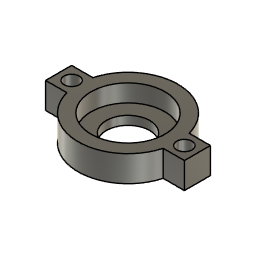
wind_direction (Autodesk Fusion 360 archive; units mm, degrees)
design "uchwyt lozysko"
Autodesk Fusion 360 part; units mm, degrees
sketch "Szkic1" plane through (0, 0, 0) normal (0, 0, 1) x (1, 0, 0)
  circle A0 centre (0, 0) radius 5
  circle A1 centre (0, 0) radius 8.5
  circle A2 centre (0, 0) radius 11.5
  circle A3 centre (13, 0) radius 1.75
  circle A4 centre (-13, 0) radius 1.75
  line L0 (16, 3) -> (-16, 3)
  line L1 (-16, 3) -> (-16, -3)
  line L2 (-16, -3) -> (16, -3)
  line L3 (16, -3) -> (16, 3)
  line L4 (16, 3) -> (-16, -3) construction
  line L5 (-16, 3) -> (16, -3) construction
  dimension "d1" = 10
  dimension "d2" = 17
  dimension "d3" = 23
  dimension "d4" = 3.5
  dimension "d5" = 13
  dimension "d6" = 3.5
  dimension "d7" = 13
  dimension "d8" = 32
  dimension "d9" = 6
  constraint coincident A0.centre A1.centre
  constraint concentric A0 A2
  constraint horizontal L0
  constraint perpendicular L0 L1
  constraint parallel L0 L2
  constraint parallel L1 L3
  constraint coincident L4 A0.centre
  constraint coincident L5 A0.centre
  constraint horizontal A0.centre A4.centre
  constraint horizontal A0.centre A3.centre
  measures "d1" diameter of A0
  measures "d2" diameter of A1
  measures "d3" diameter of A2
  measures "d4" diameter of A3
  measures "d5" distance of A0.centre A3.centre
  measures "d6" diameter of A4
  measures "d7" distance of A0.centre A4.centre
  measures "d8" distance of L1.end L2.end
  measures "d9" distance of L0.end L1.end
extrude "Wyciągnięcie proste1" add sketch "Szkic1" along normal blind 6 contours A1 A2 A3 L0 L2 | A1 A2 L0 | A1 A2 L2 | A1 A2 A4 L0 L2 | A2 A3 L0 L2 L3 | A2 A4 L0 L1 L2
extrude "Wyciągnięcie proste2" add sketch "Szkic1" along normal blind 2 contours A0 A1 L0 L2 | A0 A1 L0 | A0 A1 L2 | A0 A1 L0 L2

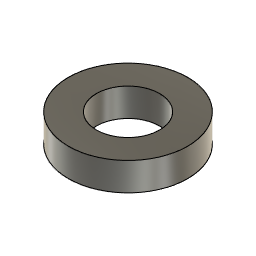
design "lozysko"
Autodesk Fusion 360 part; units mm, degrees
sketch "Szkic1" plane through (0, 0, 0) normal (0, 0, 1) x (1, 0, 0)
  circle A0 centre (0, 0) radius 4.5
  circle A1 centre (0, 0) radius 8.5
  dimension "d1" = 9
  dimension "d2" = 17
  constraint coincident A0.centre A1.centre
  constraint concentric A0 A1
  measures "d1" diameter of A0
  measures "d2" diameter of A1
extrude "Wyciągnięcie proste1" add sketch "Szkic1" along normal blind 4

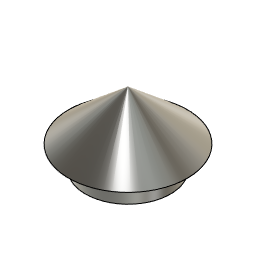
design "nakladka"
Autodesk Fusion 360 part; units mm, degrees
sketch "Szkic1" plane through (0, 0, 0) normal (0, 1, 0) x (1, 0, 0)
  line L0 (-6, 0) -> (0, -5.0346)
  line L1 (0, -3.3564) -> (0, -5.0346)
  line L2 (-2.5, 0) -> (1.3455, 0) construction
  line L3 (-2.5, 0) -> (0, -2.0977)
  line L4 (-2.5, 0) -> (1.1341, 0) construction
  line L5 (0, -2.0977) -> (0, -5.0346)
  line L6 (-2.5, 0) -> (-4, 1.2586)
  line L7 (-6, 0) -> (-4, 0) construction
  line L8 (-2.5, 0) -> (3.6054, 0) construction
  line L9 (-6, 0) -> (-8.0308, 1.704)
  line L10 (-8.0308, 1.704) -> (-6, 1.704)
  line L11 (-6, 1.704) -> (-5.75, 4.704)
  line L12 (-5.75, 4.704) -> (-4, 4.704)
  line L13 (-4, 4.704) -> (-4, 1.2586)
  dimension "d4" = 6
  dimension "d5" = 40
  dimension "d7" = 40
  dimension "d11" = 2
  dimension "d13" = 4
  dimension "d14" = 1.75
  dimension "d15" = 3
  constraint horizontal L7
  constraint perpendicular L1 L7
  constraint horizontal L2
  constraint coincident L2.start L7
  constraint horizontal L4
  constraint parallel L1 L5
  constraint parallel L3 L6
  constraint collinear L7 L8
  constraint parallel L0 L9
  constraint perpendicular L12 L13
  constraint vertical L13
  measures "d4" distance of origin L0.start
  measures "d5" angle of L0 L7
  measures "d7" angle of L3 L4
  measures "d11" horizontal distance of L6.end L10.end
  measures "d13" distance of origin L13
  measures "d14" distance of L11.end L12.end
  measures "d15" vertical distance of L10.end L11.end
revolve "Obrót1" add sketch "Szkic1" angle 360 about axis through (0, 0, 1.75) along (0, 0, 1)

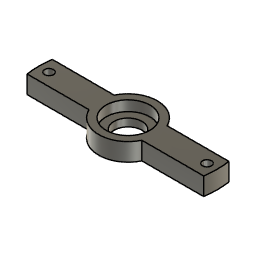
design "podstawa kierunek"
Autodesk Fusion 360 part; units mm, degrees
sketch "Szkic1" plane through (0, 0, 0) normal (0, 0, 1) x (1, 0, 0)
  circle A0 centre (0, 0) radius 11.5
  circle A1 centre (0, 0) radius 8.6
  circle A2 centre (0, 0) radius 5.5
  dimension "d1" = 23
  dimension "d2" = 17.2
  dimension "d7" = 11
  constraint coincident A0.centre A1.centre
  measures "d1" diameter of A0
  measures "d2" diameter of A1
  measures "d7" diameter of A2
extrude "Wyciągnięcie proste1" add sketch "Szkic1" along normal blind 7 contours A0
extrude "Wyciągnięcie proste2" add sketch "Szkic1" along normal blind 3 contours A1
sketch "Szkic2" plane through (0, 0, 0) normal (0, 0, 1) x (1, 0, 0)
  line L0 (13.1003, -4.95) -> (-13.365, -4.95)
  line L1 (-13.365, -4.95) -> (-13.365, 5.05)
  line L2 (-13.365, 5.05) -> (13.635, 5.05)
  line L3 (13.1003, -4.95) -> (-13.365, 5.05) construction
  line L4 (-13.365, -4.95) -> (13.635, 5.05) construction
  line L5 (35, -4.95) -> (-35, -4.95)
  line L6 (-35, -4.95) -> (-35, 4.95)
  line L7 (-35, 4.95) -> (35, 4.95)
  line L8 (35, 4.95) -> (35, -4.95)
  line L9 (35, -4.95) -> (-35, 4.95) construction
  line L10 (-13.365, -4.95) -> (-21.365, -4.95)
  line L11 (-21.365, -4.95) -> (-21.365, 4.95)
  line L12 (-21.365, 4.95) -> (-13.365, 4.95)
  line L13 (-13.365, 4.95) -> (-13.365, -4.95)
  circle A0 centre (0, 0) radius 11.5
  line L14 (-35, -4.95) -> (-11.3867, -1.6104) construction
  line L15 (0, 0) -> (35, 4.95) construction
  line L16 (-18.365, 4.95) -> (-18.365, -4.95)
  circle A1 centre (0, 0) radius 35
  circle A2 centre (-31, 0) radius 1.75
  circle A3 centre (31, 0) radius 1.75
  dimension "d8" = 27
  dimension "d9" = 10
  dimension "d10" = 70
  dimension "d11" = 9.9
  dimension "d12" = 8
  dimension "d15" = 3
  dimension "d36" = 3.5
  dimension "d37" = 4
  dimension "d38" = 4
  constraint horizontal L0
  constraint perpendicular L0 L1
  constraint parallel L0 L2
  constraint coincident L3 A0.centre
  constraint coincident L4 A0.centre
  constraint coincident A0.centre L15.start
  constraint horizontal L5
  constraint perpendicular L5 L6
  constraint parallel L5 L7
  constraint parallel L6 L8
  constraint coincident L9 A0.centre
  constraint coincident A0.centre L14
  constraint horizontal L10
  constraint vertical L11
  constraint horizontal L12
  constraint vertical L13
  constraint coincident A0 L14.end
  constraint collinear L14 L15
  constraint coincident L7 L16.start
  constraint coincident L12 L16.start
  constraint coincident L10 L16.end
  constraint coincident L5 L16.end
  constraint perpendicular L7 L16
  constraint tangent L8 A1
  constraint horizontal A0.centre A2.centre
  constraint horizontal A0.centre A3.centre
  constraint equal A2 A3
  measures "d8" distance of L1.end L2.end
  measures "d9" distance of L0.end L1.end
  measures "d10" distance of L6.end L7.end
  measures "d11" distance of L5.end L6.end
  measures "d12" distance of L0.end L10.end
  measures "d15" distance of L11 L16
  measures "d36" diameter of A3
  measures "d37" distance of L8 A3.centre
  measures "d38" distance of L6 A2.centre
extrude "Wyciągnięcie proste3" add sketch "Szkic2" along normal blind 7 contours L0 L5 L7 A0 A1 | L0 L1 L5 L7 L13 A0 | L5 L7 L11 A1 | L1 L5 L7 L10 L12 L13 L16 | L5 L7 L10 L11 L12 L16

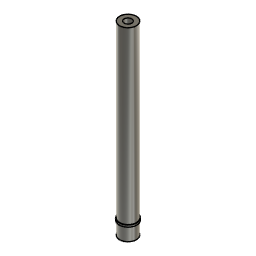
design "wal kierunek"
Autodesk Fusion 360 part; units mm, degrees
sketch "Szkic1" plane through (0, 0, 0) normal (0, 0, 1) x (1, 0, 0)
sketch "Szkic2" plane through (0, 0, 0) normal (0, 0, 1) x (1, 0, 0)
  circle A0 centre (0, 0) radius 4.5
  dimension "d1" = 9
  constraint coincident A0.centre origin
  measures "d1" diameter of A0
extrude "Wyciągnięcie proste1" add sketch "Szkic2" along normal blind 100 makes body 1
sketch "Szkic4" plane through (0, 0, 100) normal (0, 0, 1) x (-1, 0, 0)
  circle A0 centre (0, 0) radius 4.5
  circle A1 centre (0, 0) radius 2.05
  dimension "d11" = 4.1
  constraint concentric A0 A1
  measures "d11" diameter of A1
extrude "Wyciągnięcie proste4" cut sketch "Szkic4" against normal blind 8 contours A1 bodies 1
copy_body "CopyPasteBodies1" bodies 1 makes body 2
move_body "Move1" bodies 2 to x (1, 0, 0) y (0, 1, 0) z (0, 0, 1) at (50, 0, 0)
sketch "Sketch5" plane through (0, 0, 0) normal (0, 1, 0) x (1, 0, 0)
  line L0 (-40.6482, -6) -> (59.3518, -6)
  line L1 (59.3518, -6) -> (59.3518, -34)
  line L2 (59.3518, -34) -> (-40.6482, -34)
  line L3 (-40.6482, -34) -> (-40.6482, -6)
  line L4 (-40.6482, -6) -> (59.3518, -34) construction
  line L5 (59.3518, -6) -> (-40.6482, -34) construction
  point P0 (9.3518, -20)
  dimension "d14" = 100
  dimension "d15" = 28
  dimension "d46" = 20
  constraint horizontal L0
  constraint perpendicular L0 L1
  constraint parallel L0 L2
  constraint parallel L1 L3
  constraint coincident L4 P0
  constraint coincident L5 P0
  measures "d14" distance of L1.end L2.end
  measures "d15" distance of L0.end L1.end
  measures "d46" vertical distance of origin P0
extrude "Extrude5" cut sketch "Sketch5" along normal mid plane 100 bodies 1 makes body 3 at (4.4776, 0.4481, 56)
sketch "Sketch6" plane through (0, 0, 6) normal (0, 0, 1) x (-1, 0, 0)
  circle A0 centre (0, 0) radius 4.5
  circle A1 centre (0, 0) radius 3
  dimension "d18" = 6
  constraint concentric A0 A1
  measures "d18" diameter of A1
extrude "Extrude6" cut sketch "Sketch6" against normal blind 20 contours A1 bodies 1
sketch "Sketch7" plane through (0, 0, 6) normal (0, 0, 1) x (-1, 0, 0)
  circle A0 centre (0, 0) radius 3
  circle A1 centre (0, 0) radius 4.5
  line L0 (15, 15) -> (-15, 15)
  line L1 (-15, 15) -> (-15, -15)
  line L2 (-15, -15) -> (15, -15)
  line L3 (15, -15) -> (15, 15)
  line L4 (15, 15) -> (-15, -15) construction
  line L5 (-15, 15) -> (15, -15) construction
  circle A2 centre (0, 0) radius 3
  circle A3 centre (0, 0) radius 8.5
  line L6 (0, 0) -> (-6, 0)
  dimension "d21" = 30
  dimension "d22" = 30
  dimension "d33" = 17
  constraint horizontal L0
  constraint perpendicular L0 L1
  constraint parallel L0 L2
  constraint parallel L1 L3
  constraint coincident L4 A0.centre
  constraint coincident L5 A0.centre
  constraint coincident A0.centre A1.centre
  constraint horizontal L6
  measures "d21" distance of L1.end L2.end
  measures "d22" distance of L0.end L1.end
  measures "d33" diameter of A3
extrude "Extrude7" add sketch "Sketch7" along normal blind 2 contours A1 | L0 L1 L2 L3 | A3 bodies 1
sketch "Sketch8" plane through (0, 0, 34) normal (0, 0, -1) x (1, 0, 0)
  circle A0 centre (0, 0) radius 4.5
  line L0 (15, -15) -> (-15, -15)
  line L1 (-15, -15) -> (-15, 15)
  line L2 (-15, 15) -> (15, 15)
  line L3 (15, 15) -> (15, -15)
  constraint horizontal L0
  constraint vertical L1
  constraint horizontal L2
  constraint vertical L3
extrude "Extrude8" add sketch "Sketch8" along normal blind 2 separate body contours A0 | L0 L1 L2 L3 makes body 4
sketch "Sketch9" plane through (0, 0, 8) normal (0, 0, 1) x (-1, 0, 0)
  circle A0 centre (0, 0) radius 3
  line L0 (15, -15) -> (15, 15)
  line L1 (15, 15) -> (-15, 15)
  line L2 (-15, 15) -> (-15, -15)
  line L3 (-15, -15) -> (15, -15)
  line L4 (-15, 15) -> (-11, 15)
  line L5 (-11, 15) -> (-11, 11)
  line L6 (-11, 11) -> (-15, 11)
  line L7 (-15, 11) -> (-15, 15)
  line L8 (15, 15) -> (11, 15)
  line L9 (11, 15) -> (11, 11)
  line L10 (11, 11) -> (15, 11)
  line L11 (15, 11) -> (15, 15)
  line L12 (-15, -15) -> (-11, -15)
  line L13 (-11, -15) -> (-11, -11)
  line L14 (-11, -11) -> (-15, -11)
  line L15 (-15, -11) -> (-15, -15)
  circle A1 centre (0, 0) radius 8.5
  circle A2 centre (0, 0) radius 11.5
  line L16 (0, 0) -> (-8.1317, -8.1317)
  line L17 (0, 0) -> (11.5, 0) construction
  line L18 (0, 0) -> (8.1317, -8.1317)
  line L19 (0, 0) -> (11.5, 0) construction
  line L20 (15, -15) -> (11, -15)
  line L21 (11, -15) -> (11, -11)
  line L22 (11, -11) -> (15, -11)
  line L23 (15, -11) -> (15, -15)
  line L24 (-11, -11) -> (-11, 11)
  dimension "d29" = 17
  dimension "d30" = 23
  dimension "d31" = 135
  dimension "d32" = 45
  constraint horizontal L4
  constraint vertical L5
  constraint horizontal L6
  constraint vertical L7
  constraint coincident L1.end L2.start
  constraint horizontal L8
  constraint vertical L9
  constraint horizontal L10
  constraint vertical L11
  constraint coincident L0.end L1.start
  constraint horizontal L12
  constraint vertical L13
  constraint horizontal L14
  constraint vertical L15
  constraint coincident L2.end L3.start
  constraint coincident A0.centre A1.centre
  constraint concentric A1 A2
  constraint horizontal L17
  constraint horizontal L19
  constraint horizontal L20
  constraint vertical L21
  constraint horizontal L22
  constraint vertical L23
  constraint coincident L0.start L3.end
  constraint equal L8 L22
  constraint equal L9 L21
  constraint perpendicular L6 L24
  constraint coincident A2 L16.end
  measures "d29" diameter of A1
  measures "d30" diameter of A2
  measures "d31" angle of L16 L17
  measures "d32" angle of L18 L19
extrude "Extrude9" add sketch "Sketch9" along normal up to surface (24 mm away) contours A1 A2 L16 L18 | L2 L6 L14 A2 L24 | L2 L3 L12 L13 L14 L15 | L1 L2 L4 L5 L6 L7 | L0 L3 L20 L21 L22 L23 | L0 L1 L8 L9 L10 L11 bodies 1 4
sketch "Sketch11" plane through (0, 0, 32) normal (0, 0, -1) x (1, 0, 0)
  line L0 (-11, -11) -> (-11, -15)
  line L1 (-11, -15) -> (11, -15)
  line L2 (11, -15) -> (11, -3.3541)
  arc A0 (11, -3.3541) -> (11, 3.3541) centre (0, 0) ccw
  line L3 (11, 3.3541) -> (11, 15)
  line L4 (11, 15) -> (-11, 15)
  line L5 (-11, 15) -> (-11, 11)
  line L6 (-11, 11) -> (-15, 11)
  line L7 (-15, 11) -> (-15, -11)
  line L8 (-15, -11) -> (-11, -11)
  arc A1 (-8.1317, -8.1317) -> (8.1317, -8.1317) centre (0, 0) ccw
  line L9 (-8.1317, -8.1317) -> (-6.0104, -6.0104)
  arc A2 (-6.0104, -6.0104) -> (6.0104, -6.0104) centre (0, 0) ccw
  line L10 (6.0104, -6.0104) -> (8.1317, -8.1317)
  line L11 (11, -15) -> (-11, -15)
  line L12 (-11, -15) -> (-11, -11)
  line L13 (-11, -11) -> (11, -11)
  line L14 (11, -11) -> (11, -15)
  line L15 (-11, -11) -> (-15, -11)
  line L16 (-15, -11) -> (-15, 11)
  line L17 (-15, 11) -> (-11, 11)
  line L18 (-11, 11) -> (-11, -11)
  line L19 (-11, 11) -> (11, 11)
  line L20 (11, 11) -> (11, 15)
  line L21 (11, 15) -> (-11, 15)
  line L22 (-11, 15) -> (-11, 11)
  constraint horizontal L11
  constraint vertical L12
  constraint horizontal L13
  constraint vertical L14
  constraint coincident L0.start L8.end
  constraint coincident L1.end L2.start
  constraint horizontal L15
  constraint vertical L16
  constraint horizontal L17
  constraint vertical L18
  constraint coincident L6.end L7.start
  constraint horizontal L19
  constraint vertical L20
  constraint horizontal L21
  constraint vertical L22
  constraint coincident L3.end L4.start
  constraint coincident L5.end L6.start
extrude "Extrude12" add sketch "Sketch11" along normal blind 0.4 contours L0 L1 L2 A1 L11 L12 L13 L14 | L6 L7 L8 L15 L16 L17 L18 | L3 L4 L5 L19 L20 L21 L22 bodies 1
draft "Draft1" angle 1 neutral plane through (0, 0, 0) pull (0, 0, -1) 1 faces at (4.4776, 0.4481, 4) on bodies 1
sketch "Sketch12" plane through (0, 0, 8) normal (0, 0, 1) x (-1, 0, 0)
  circle A0 centre (0, 0) radius 3
  line L0 (11, -15) -> (11, -11)
  line L1 (11, -11) -> (15, -11)
  line L2 (15, -11) -> (15, 11)
  line L3 (15, 11) -> (11, 11)
  line L4 (11, 11) -> (11, 15)
  line L5 (11, 15) -> (-11, 15)
  line L6 (-11, 15) -> (-11, 3.3541)
  arc A1 (-11, 3.3541) -> (-11, -3.3541) centre (0, 0) ccw
  line L7 (-11, -3.3541) -> (-11, -15)
  line L8 (-11, -15) -> (11, -15)
  arc A2 (-8.1317, -8.1317) -> (8.1317, -8.1317) centre (0, 0) ccw
  line L9 (-8.1317, -8.1317) -> (-6.0104, -6.0104)
  arc A3 (-6.0104, -6.0104) -> (6.0104, -6.0104) centre (0, 0) ccw
  line L10 (6.0104, -6.0104) -> (8.1317, -8.1317)
  line L11 (2.5, 15) -> (-2.5, 15)
  line L12 (-2.5, 15) -> (-2.5, 0)
  line L13 (-2.5, 0) -> (2.5, 0)
  line L14 (2.5, 0) -> (2.5, 15)
  dimension "d55" = 5
  dimension "d56" = 15
  dimension "d57" = 2.5
  constraint horizontal L11
  constraint vertical L12
  constraint horizontal L13
  constraint vertical L14
  constraint coincident L5 L11.start
  measures "d55" distance of L11.start L11.end
  measures "d56" distance of L11.start L13.end
  measures "d57" distance of A0.centre L12
extrude "Extrude13" cut sketch "Sketch12" against normal blind 4 contours A0 L5 L11 L12 L14 bodies 1
fillet "Fillet1" radius 2 1 edges at (0, -3, 4) on bodies 1
ref_plane "WorkPlane1" through (50, 0, 7) normal (0, 0, -1) x (-1, 0, 0)
sketch "Sketch13" plane through (0, 0, 7) normal (0, 0, -1) x (-1, 0, 0)
  circle A0 centre (-50, 0) radius 4.75
  circle A1 centre (-50, 0) radius 2.05
  dimension "d63" = 9.5
  constraint concentric A0 A1
  measures "d63" diameter of A0
extrude "Extrude14" add sketch "Sketch13" against normal blind 1 bodies 2
sketch "Sketch14" plane through (0, 0, 0) normal (0, 0, -1) x (1, 0, 0)
  circle A0 centre (50, 0) radius 4.5
  circle A1 centre (50, 0) radius 2
  dimension "d66" = 4
  constraint concentric A0 A1
  measures "d66" diameter of A1
extrude "Extrude15" cut sketch "Sketch14" against normal blind 2 contours A1 bodies 2
hidden bodies 1 3
named bodies: "new_shaft"
